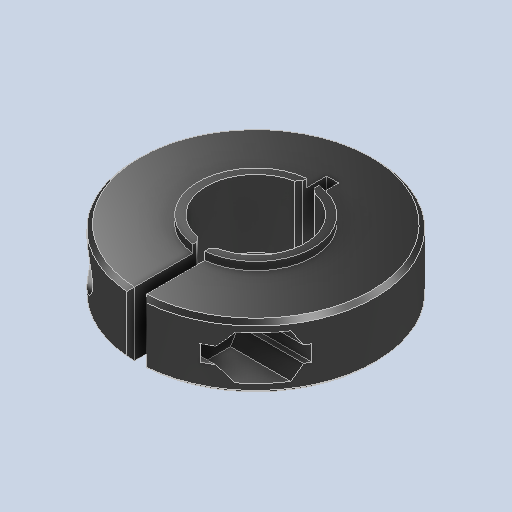
# Autodesk Inventor part: omu_3d_jo_1
Saved by Autodesk Inventor 2025.1 (Build 291241000, 241)
## iProperties
Created: 2023-11-22
Part Number: omu_3d_jo_1
Material: ABS プラスチック
Document SubType Name: Modeling
Designer: fhbdh
Density: 1.06 g/cm^3
Appearance: 光沢 - 黒
Author: fhbdh
Autodesk Inventor part; units mm, degrees
sketch "スケッチ1" plane through (0, 0, 0) normal (0, 1, 0) x (-1, 0, 0)
  circle A0 centre (0, 0) radius 6.2
  circle A1 centre (0, 0) radius 15
  line L0 (0, 15) -> (0, 0) construction
  line L1 (0.75, 14.9812) -> (0.75, 6.1545)
  line L2 (-0.75, 14.9812) -> (-0.75, 6.1545)
  line L3 (0.75, -6.1545) -> (0.75, -9.6545)
  line L4 (0.75, -9.6545) -> (-0.75, -9.6545)
  line L5 (-0.75, -9.6545) -> (-0.75, -6.1545)
  line L6 (0, 0) -> (15, 0) construction
  dimension "d0" = 12.4
  dimension "d1" = 30
  dimension "d2" = 1.5
  dimension "d3" = 1.5
  dimension "d4" = 3.5
  constraints: 14 end point, 8 point on circle, 3 vertical, 2 centre point, 2 coincident, 2 perpendicular, 1 horizontal, 1 parallel, 2 other
  measures "d0" diameter of A0
  measures "d1" diameter of A1
  measures "d2" distance between parallel lines of L2 L1
  measures "d3" distance of L3.end L4.end
  measures "d4" distance of L4.end L5.end
extrude "押し出し1" add sketch "スケッチ1" along normal blind 8 contours A0 L1 A1 L2 L5 L4 L3
ref_plane "作業平面1" through (-15, 0, 0) normal (1, 0, 0) x (0, 1, 0)
sketch "スケッチ2" plane through (-15, 0, 0) normal (1, 0, 0) x (0, 1, 0)
  circle A0 centre (4, 9.9906) radius 1.5
  line L0 (8, -15) -> (8, 14.9812) projected
  line L1 (0, -15) -> (0, 14.9812) projected
  point P0 (0, 0)
  point P1 (0, -0.0094)
  dimension "d13" = 3
  dimension "d14" = 8
  dimension "d15" = 4
  dimension "d16" = 10
  constraints: 1 centre point, 1 midpoint
  measures "d13" diameter of A0
  measures "d14" distance between parallel lines of L0 L1
  measures "d15" distance from line of L1 A0.centre
  measures "d16" vertical distance of point (0, -0.009) A0.centre
extrude "押し出し2" cut sketch "スケッチ2" along normal through all
sketch "スケッチ3" plane through (0, 0, 0) normal (1, 0, 0) x (0, 1, 0)
  line L0 (0, -15) -> (0, 14.9812) projected
  line L1 (8, -15) -> (8, 14.9812) projected
  point P0 (0, 0)
  dimension "d19" = 8
  measures "d19" distance between parallel lines of L0 L1
ref_plane "作業平面2" through (0, 4, 0) normal (0, -1, 0) x (1, 0, 0)
sketch "スケッチ4" plane through (0, 4, 0) normal (0, -1, 0) x (1, 0, 0)
  line L0 (-9.6419, 11.4906) -> (-0.75, 11.4906) projected
  point P0 (0, 0)
ref_plane "作業平面3" through (-9.6419, 4, 11.4906) normal (1, 0, 0) x (0, 1, 0)
sketch "スケッチ6" plane through (-9.6419, 4, 11.4906) normal (1, 0, 0) x (0, 1, 0)
  spline S0 degree 2 poles (1.5, -1.5) (1.5, -4.0981) (-0.75, -2.799) (-3, -1.5) (-0.75, -0.201) (1.5, 1.0981) (1.5, -1.5) knots 0 0 0 0.333333 0.333333 0.666667 0.666667 1 1 1 weights 1 0.5 1 0.5 1 0.5 1 projected
  circle A0 centre (0, -1.5) radius 3
  circle A1 centre (0, -1.5) radius 1.5 projected
  line L0 (-1.5, -1.5) -> (0, -1.5) construction
  point P0 (-4, -11.4906)
  dimension "d21" = 6
  constraints: 2 end point, 1 centre point, 1 coincident, 1 horizontal, 1 point on circle, 2 other
  measures "d21" diameter of A0
extrude "押し出し3" cut sketch "スケッチ6" along normal blind 5 and the other way blind 10
ref_plane "作業平面4" through (15, 0, 0) normal (1, 0, 0) x (0, 1, 0)
sketch "スケッチ7" plane through (15, 0, 0) normal (1, 0, 0) x (0, 1, 0)
  spline S0 degree 2 poles (5.5, 9.9906) (5.5, 7.3925) (3.25, 8.6916) (1, 9.9906) (3.25, 11.2897) (5.5, 12.5887) (5.5, 9.9906) knots 0 0 0 0.333333 0.333333 0.666667 0.666667 1 1 1 weights 1 0.5 1 0.5 1 0.5 1 projected
  circle A0 centre (4, 9.9906) radius 1.5 projected
  line L0 (5.5, 9.9906) -> (4, 9.9906) construction
  line L1 (1.25, 6.4906) -> (6.75, 6.4906)
  line L2 (6.75, 6.4906) -> (6.75, 13.4906)
  line L3 (6.75, 13.4906) -> (1.25, 13.4906)
  line L4 (1.25, 13.4906) -> (1.25, 6.4906)
  line L5 (1.25, 6.4906) -> (6.75, 13.4906) construction
  line L6 (6.75, 6.4906) -> (1.25, 13.4906) construction
  line L7 (6.95, 11.6938) -> (6.95, 8.2874)
  line L8 (6.95, 8.2874) -> (4, 6.5843)
  line L9 (4, 6.5843) -> (1.05, 8.2874)
  line L10 (1.05, 8.2874) -> (1.05, 11.6938)
  line L11 (1.05, 11.6938) -> (4, 13.397)
  line L12 (4, 13.397) -> (6.95, 11.6938)
  line L13 (5, 13.4906) -> (5, 12.8196)
  line L14 (3, 13.4906) -> (3, 12.8196)
  line L15 (5, 7.1616) -> (5, 6.4906)
  line L16 (3, 7.1616) -> (3, 6.4906)
  line L17 (4, 11.4906) -> (4, 8.4906) construction
  point P0 (0, 0)
  point P1 (1.25, 11.8093)
  point P2 (1.25, 8.172)
  point P3 (6.75, 8.172)
  point P4 (6.75, 11.8093)
  dimension "d26" = 7
  dimension "d27" = 5.5
  dimension "d36" = 5.9
  dimension "d37" = 2
  dimension "d38" = 2
  constraints: 36 end point, 8 point on line, 4 parallel, 3 midpoint, 3 perpendicular, 2 horizontal, 2 vertical, 1 coincident, 1 point on circle, 18 other
  measures "d26" distance of L1.end L2.end
  measures "d27" distance of L2.end L3.end
  measures "d36" distance between parallel lines of L9 L12
  measures "d37" distance between parallel lines of L14 L13
  measures "d38" distance between parallel lines of L15 L16
extrude "押し出し4" cut sketch "スケッチ7" against normal blind 10 contours L16 L9 L8 L15 L1 | L4 L11 L12 L2 L8 L9 | L14 L3 L13 L12 L11
sketch "スケッチ8" plane through (0, 8, 0) normal (0, 1, 0) x (1, 0, 0)
  circle A0 centre (0, 0) radius 7.2
  arc A1 (-0.75, 6.1545) -> (-0.75, -6.1545) centre (0, 0) ccw projected
  line L0 (-0.75, 6.1545) -> (-0.75, 9.6545) projected
  line L1 (0.75, 9.6545) -> (0.75, 6.1545) projected
  arc A2 (0.75, -6.1545) -> (0.75, 6.1545) centre (0, 0) ccw projected
  line L2 (0.75, -6.1545) -> (0.75, -14.9812) projected
  line L3 (-0.75, -14.9812) -> (-0.75, -6.1545) projected
  point P0 (0.75, -7.1608)
  point P1 (0.75, 7.1608)
  point P2 (-0.75, 7.1608)
  point P3 (-0.75, -7.1608)
  dimension "d39" = 1
  constraints: 1 centre point, 1 coincident
  measures "d39" radial gap between concentric circles of A0 A1
extrude "押し出し5" add sketch "スケッチ8" along normal blind 1 contours A0 L2 A2 L1 | L0 A1 L3 A0
chamfer "面取り3" distance 0.5 angle 45 10 edges at (0, 0, -15) (-6.2, 0, 0) (6.2, 0, 0) (0.75, 4, 14.9812) (-0.75, 4, 14.9812) (0, 8, -15) (0.75, 4.5, 6.1545) (-0.75, 4.5, 6.1545) (-0.75, 4.5, -6.1545) (0.75, 4.5, -6.1545)
equation "\"d3\" = d2"
equation "\"d15\" = 0.5 * d14"
equation "\"d38\" = d37"
equation "\"d20\" = -0.5 * d19"
